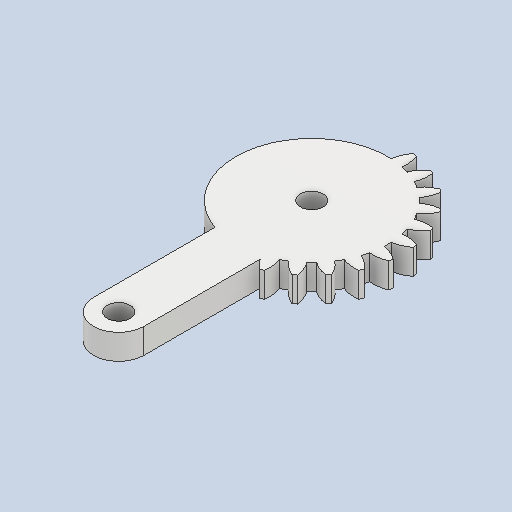
# Autodesk Inventor part: zubate_kolo1
Saved by Autodesk Inventor 2023 (Build 270158000, 158)
## iProperties
Part Number: zubate_kolo1
Material: ABS Plastic
Document SubType Name: Modeling
Designer: denyh
Density: 1.06 g/cm^3
Appearance: Smooth - White
Mass: 2.7921 g
Surface Area: 20.5354 cm^2
Volume: 2.63405 cm^3
Author: denyh
Autodesk Inventor part; units mm, degrees
ref_plane "YZ Plane" through (0, 0, 0) normal (1, 0, 0) x (0, 1, 0)
ref_plane "XZ Plane" through (0, 0, 0) normal (0, 1, 0) x (-1, 0, 0)
ref_plane "XY Plane" through (0, 0, 0) normal (0, 0, 1) x (1, 0, 0)
sketch "Náčrt1" plane through (0, 0, 0) normal (0, 0, 1) x (1, 0, 0)
  circle A0 centre (0, 0) radius 12.093
  circle A1 centre (0, 0) radius 1.825
  dimension "d0" = 24.186
  dimension "d1" = 3.65
  constraints: 2 centre point, 2 coincident
  measures "d0" diameter of A0
  measures "d1" diameter of A1
extrude "Vysunutí1" add sketch "Náčrt1" along normal blind 4
sketch "Náčrt2" plane through (0, 0, 0) normal (0, 0, -1) x (-1, 0, 0)
  line L0 (0, 0) -> (0, 17.286)
  circle A0 centre (0, 0) radius 1.825 projected
  line L1 (0, 0) -> (3.0566, 13.6745)
  line L2 (0, 0) -> (-0.9214, -21.9835)
  arc A1 (-0.5405, 12.0809) -> (-1.5985, 14.5344) centre (-5.8739, 11.2357) ccw
  arc A2 (-8.6515, 11.7879) -> (-9.147, 11.4077) centre (0, 0) ccw
  arc A3 (-11.4077, 9.147) -> (-11.7879, 8.6515) centre (0, 0) ccw
  arc A4 (-5.3058, 13.6254) -> (-5.8828, 13.3864) centre (0, 0) ccw
  arc A5 (-13.3864, 5.8828) -> (-13.6254, 5.3058) centre (0, 0) ccw
  arc A6 (-14.4528, 2.2177) -> (-14.5344, 1.5985) centre (0, 0) ccw
  arc A7 (-14.5344, -1.5985) -> (-14.4528, -2.2177) centre (0, 0) ccw
  arc A8 (-13.6254, -5.3058) -> (-13.3864, -5.8828) centre (0, 0) ccw
  arc A9 (-11.7879, -8.6515) -> (-11.4077, -9.147) centre (0, 0) ccw
  arc A10 (-9.147, -11.4077) -> (-8.6515, -11.7879) centre (0, 0) ccw
  arc A11 (-5.8828, -13.3864) -> (-5.3058, -13.6254) centre (0, 0) ccw
  arc A12 (-1.5985, 14.5344) -> (-2.2177, 14.4528) centre (0, 0) ccw
  circle A13 centre (0, 0) radius 12.093 projected
  arc A14 (-2.2177, 14.4528) -> (-2.6047, 11.8091) centre (2.7657, 12.3732) ccw
  arc A15 (-5.8828, 13.3864) -> (-5.5724, 10.7326) centre (-0.5309, 12.6674) ccw
  arc A16 (-9.147, 11.4077) -> (-8.1603, 8.9247) centre (-3.7914, 12.0983) ccw
  arc A17 (-11.7879, 8.6515) -> (-10.1922, 6.5085) centre (-6.7935, 10.7048) ccw
  arc A18 (-13.6254, 5.3058) -> (-11.5294, 3.6488) centre (-9.3326, 8.5818) ccw
  arc A19 (-14.5344, 1.5985) -> (-12.0809, 0.5405) centre (-11.2357, 5.8739) ccw
  arc A20 (-14.4528, -2.2177) -> (-11.8091, -2.6047) centre (-12.3732, 2.7657) ccw
  arc A21 (-13.3864, -5.8828) -> (-10.7326, -5.5724) centre (-12.6674, -0.5309) ccw
  arc A22 (-11.4077, -9.147) -> (-8.9247, -8.1603) centre (-12.0983, -3.7914) ccw
  arc A23 (-8.6515, -11.7879) -> (-6.5085, -10.1922) centre (-10.7048, -6.7935) ccw
  arc A24 (-5.3058, -13.6254) -> (-3.6488, -11.5294) centre (-8.5818, -9.3326) ccw
  arc A25 (-3.6488, 11.5294) -> (-5.3058, 13.6254) centre (-8.5818, 9.3326) ccw
  arc A26 (-6.5085, 10.1922) -> (-8.6515, 11.7879) centre (-10.7048, 6.7935) ccw
  arc A27 (-8.9247, 8.1603) -> (-11.4077, 9.147) centre (-12.0983, 3.7914) ccw
  arc A28 (-10.7326, 5.5724) -> (-13.3864, 5.8828) centre (-12.6674, 0.5309) ccw
  arc A29 (-11.8091, 2.6047) -> (-14.4528, 2.2177) centre (-12.3732, -2.7657) ccw
  arc A30 (-12.0809, -0.5405) -> (-14.5344, -1.5985) centre (-11.2357, -5.8739) ccw
  arc A31 (-11.5294, -3.6488) -> (-13.6254, -5.3058) centre (-9.3326, -8.5818) ccw
  arc A32 (-10.1922, -6.5085) -> (-11.7879, -8.6515) centre (-6.7935, -10.7048) ccw
  arc A33 (-8.1603, -8.9247) -> (-9.147, -11.4077) centre (-3.7914, -12.0983) ccw
  arc A34 (-5.5724, -10.7326) -> (-5.8828, -13.3864) centre (-0.5309, -12.6674) ccw
  dimension "d6" = 12.6
  dimension "d17" = 169.8
  dimension "d22" = 10.8
  dimension "d29" = 150
  dimension "d33" = 150
  constraints: 68 point on circle, 33 centre point, 6 end point, 2 coincident, 1 point on line, 1 vertical, 82 other
  measures "d6" angle of L0 L1
  measures "d17" angle of L1 L2
  measures "d22" diameter of A1
extrude "Vysunutí2" add sketch "Náčrt2" against normal blind 4 contours A13 A14 A12 A1
pattern_circular "Kruhové pole1" count 11 over 150 about axis through (0, 0, 0) along (0, 0, -1) of "Vysunutí2"
sketch "Náčrt3" plane through (0, 0, 4) normal (0, 0, 1) x (1, 0, 0)
  line L0 (0, 0) -> (0, -30.722)
  circle A0 centre (0, -30.722) radius 1.825
  line L1 (-4, 1.3777) -> (-4, -30.722)
  line L2 (4, 1.3777) -> (4, -30.722)
  arc A1 (-4, -30.722) -> (4, -30.722) centre (0, -30.722) ccw
  line L3 (-4, -8.9953) -> (4, -8.9953)
  point P0 (-4, -33.1583)
  point P1 (4, -33.1583)
  dimension "d40" = 30.722
  dimension "d41" = 3.65
  dimension "d42" = 34.536
  dimension "d43" = 4
  dimension "d44" = 8
  constraints: 8 end point, 2 centre point, 2 coincident, 2 point on circle, 2 point on line, 2 symmetric about line, 2 vertical, 1 perpendicular
  measures "d40" distance of L0.start L0.end
  measures "d41" diameter of A0
  measures "d42" distance of L1.start point (-4, -33.158)
  measures "d43" distance between parallel lines of L0 L1
  measures "d44" diameter of A1
extrude "Vysunutí3" add sketch "Náčrt3" against normal blind 4
